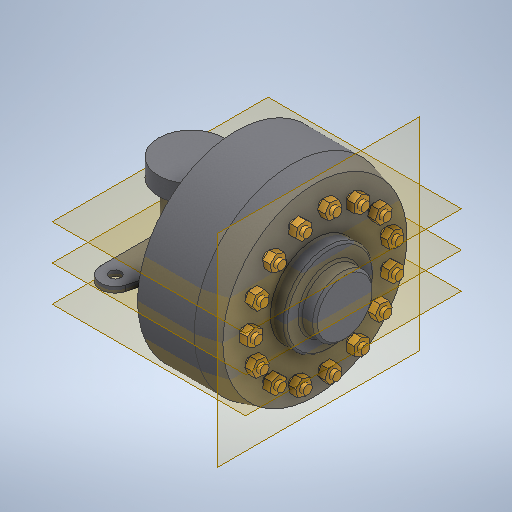
# Autodesk Inventor part: eg 243 hub 2nd ver
Saved by Autodesk Inventor 2025 (Build 290162000, 162)
## iProperties
Created: 2024-11-03
Part Number: eg 243 hub 2nd ver
Material: Generic
Document SubType Name: Modeling
Designer: Student
Density: 1 g/cm^3
Appearance: Default
Author: Student
Autodesk Inventor part; units mm, degrees
ref_plane "YZ Plane" through (0, 0, 0) normal (1, 0, 0) x (0, 1, 0)
ref_plane "XY Plane" through (0, 0, 0) normal (0, 0, 1) x (1, 0, 0)
sketch "Sketch1" plane through (0, 0, 0) normal (0, 0, 1) x (1, 0, 0)
  line L0 (0, 0) -> (0, 165)
  line L1 (0, 165) -> (95, 165)
  line L2 (95, 165) -> (133, 154.8179)
  line L3 (133, 154.8179) -> (133, 75)
  line L4 (133, 75) -> (158, 75)
  line L5 (158, 75) -> (158, 50)
  line L6 (158, 50) -> (183, 50)
  line L7 (183, 50) -> (183, 0)
  line L8 (183, 0) -> (0, 0)
  point P0 (0, 0)
  dimension "d0" = 165
  dimension "d1" = 95
  dimension "d2" = 38
  dimension "d3" = 15
  dimension "d4" = 25
  dimension "d5" = 25
  dimension "d6" = 25
  dimension "d7" = 50
  dimension "d8" = 0
  dimension "d9" = 0
  constraints: 18 end point, 5 perpendicular, 1 horizontal, 1 parallel, 1 vertical
  measures "d0" distance of L0.start L0.end
  measures "d1" distance of L0.end L1.end
  measures "d2" distance from line of L3 L1.end
  measures "d3" angle of L1 L2
  measures "d4" distance of L3.end L4.end
  measures "d5" distance of L4.end L5.end
  measures "d6" distance of L5.end L6.end
  measures "d7" distance of L6.end L7.end
  measures "d8" distance from line of L8 point (0, 0)
  measures "d9" distance from line of L0 point (0, 0)
revolve "Revolution1" add sketch "Sketch1" angle 360 about axis through (183, 0, 0) along (-1, 0, 0)
chamfer "Chamfer1" distance 4 angle 45 1 edges at (183, -50, 0)
fillet "Fillet1" radius 3.5 1 edges at (158, -50, 0)
fillet "Fillet2" radius 3.5 1 edges at (158, -75, 0)
sketch "Sketch2" plane through (0, 0, 0) normal (0, 1, 0) x (-1, 0, 0)
  circle A0 centre (75, 0) radius 37.5
  line L0 (0, -165) -> (0, 165) projected
  point P0 (0, 0)
  dimension "d16" = 75
  dimension "d17" = 75
  constraints: 1 centre point
  measures "d16" distance from line of A0.centre L0
  measures "d17" diameter of A0
extrude "Extrusion1" add sketch "Sketch2" along normal blind 90 and the other way blind 80
sketch "Sketch3" plane through (0, 0, 0) normal (0, 1, 0) x (-1, 0, 0)
  circle A0 centre (75, 0) radius 37.5 projected
  line L0 (0, 0) -> (0, 50)
  line L1 (0, -165) -> (0, 165) projected
  line L2 (0, 50) -> (25, 50)
  line L3 (25, 50) -> (83.418, 36.543)
  line L4 (0, 0) -> (0, -50)
  line L5 (0, -50) -> (25, -50)
  line L6 (25, -50) -> (83.418, -36.543)
  dimension "d22" = 50
  dimension "d23" = 25
  constraints: 12 end point, 1 horizontal, 1 point on line, 3 other
  measures "d22" distance of L0.start L0.end
  measures "d23" distance of L0.end L2.end
ref_plane "Work Plane1" through (0, 60, 0) normal (0, 1, 0) x (-1, 0, 0)
ref_plane "Work Plane2" through (0, -60, 0) normal (0, 1, 0) x (-1, 0, 0)
extrude "Extrusion2" add sketch "Sketch3" along normal blind 12.5 from surface at -60 contours A0 L6 L5 L1 L0 L2 L3
ref_plane "Work Plane3" through (0, 0, 0) normal (0, 1, 0) x (-1, 0, 0)
mirror "Mirror1" about plane through (0, 0, 0) normal (0, 1, 0) of "Extrusion2"
sketch "Sketch4" plane through (0, 0, 0) normal (0, 1, 0) x (-1, 0, 0)
  line L0 (0, -165) -> (0, 165) projected
  line L1 (0, 50) -> (0, -100)
  line L2 (0, -100) -> (25, -100)
  line L3 (77.733, 0) -> (77.733, -37.4003)
  line L4 (77.733, 0) -> (77.733, 40.4043)
  circle A0 centre (75, 0) radius 37.5 projected
  line L5 (77.733, -37.4003) -> (25, -100)
  line L6 (77.733, 37.4003) -> (77.733, 150)
  line L7 (0, -100) -> (0, 50)
  line L8 (0, 50) -> (28.588, 156.4824)
  arc A1 (77.733, 150) -> (28.588, 156.4824) centre (52.733, 150) ccw
  circle A2 centre (52.733, 150) radius 9.5
  point P0 (0, 0)
  point P1 (0, 50)
  dimension "d29" = 0
  dimension "d30" = 150
  dimension "d31" = 25
  dimension "d32" = 100
  dimension "d33" = 150
  dimension "d34" = 25
  dimension "d35" = 19
  constraints: 16 end point, 4 point on circle, 4 point on line, 2 centre point, 2 tangent, 2 vertical, 1 coincident, 1 collinear, 1 horizontal
  measures "d29" distance of point (0, 50) L1.start
  measures "d30" distance of L1.end L1.start
  measures "d31" distance of L1.end L2.end
  measures "d32" distance from line of L2 L3.start
  measures "d33" distance of L6.end L3.start
  measures "d34" radius of A1
  measures "d35" diameter of A2
extrude "Extrusion3" add sketch "Sketch4" along normal mid plane 9.5 contours L0 L8 A1 L6 L4 A0 L5 L2
sketch "Sketch5" plane through (-25, 60, 50) normal (0, 1, 0) x (1, 0, 0)
  circle A0 centre (-50, 50) radius 37.5 projected
  circle A1 centre (-50, 50) radius 55
  point P0 (25, 50)
  dimension "d38" = 110
  constraints: 1 centre point, 1 coincident
  measures "d38" diameter of A1
extrude "Extrusion4" add sketch "Sketch5" along normal up to surface (30 mm away) contours A0 | A1
sketch "Sketch6" plane through (133, 0, 0) normal (1, 0, 0) x (0, 0, -1)
  line L0 (-107.5, -7.2169) -> (-120, -14.4338)
  line L1 (-120, -14.4338) -> (-132.5, -7.2169)
  line L2 (-132.5, -7.2169) -> (-132.5, 7.2169)
  line L3 (-132.5, 7.2169) -> (-120, 14.4338)
  line L4 (-120, 14.4338) -> (-107.5, 7.2169)
  line L5 (-107.5, 7.2169) -> (-107.5, -7.2169)
  circle A0 centre (-120, 0) radius 7.5
  circle A1 centre (0, 0) radius 46 projected
  point P0 (0, 0)
  dimension "d41" = 25
  dimension "d42" = 15
  dimension "d43" = 120
  constraints: 12 end point, 1 centre point, 1 coincident, 13 other
  measures "d41" distance between parallel lines of L5 L2
  measures "d42" diameter of A0
  measures "d43" distance of A1.centre point (-120, 0)
ref_plane "Work Plane4" through (139, 0, 0) normal (1, 0, 0) x (0, 0, -1)
extrude "Extrusion5" add sketch "Sketch6" along normal blind 12.5 from surface at 6 contours L0 L1 L2 L3 L4 L5
sketch "Sketch7" plane through (133, 0, 0) normal (1, 0, 0) x (0, 0, -1)
  circle A0 centre (-120, 0) radius 7.5 projected
  circle A1 centre (-120, 0) radius 7.5
  point P0 (0, 0)
  constraints: 1 centre point, 1 coincident
extrude "Extrusion6" add sketch "Sketch7" along normal blind 25
pattern_circular "Circular Pattern1" count 15 over 360 about axis through (47.5, 0, 0) along (-1, 0, 0) of "Extrusion5", "Extrusion6"
body "Solid1"
